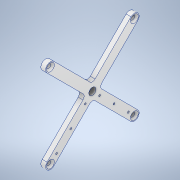
# Autodesk Inventor part: winch_support
Saved by Autodesk Inventor 2020.2 (Build 242310000, 310)
## iProperties
Created: 2020-03-23
Part Number: winch_support
Material: Aluminum 6061
Document SubType Name: Modeling
Designer: agmle
Density: 2.7 g/cm^3
Appearance: Aluminum - Flat
Mass: 66.4597 g
Surface Area: 128.224 cm^2
Volume: 24.6147 cm^3
Author: agmle
Autodesk Inventor part; units mm, degrees
ref_plane "YZ Plane" through (0, 0, 0) normal (1, 0, 0) x (0, 1, 0)
ref_plane "XZ Plane" through (0, 0, 0) normal (0, 1, 0) x (-1, 0, 0)
ref_plane "XY Plane" through (0, 0, 0) normal (0, 0, 1) x (1, 0, 0)
sketch "Sketch1" plane through (0, 0, 0) normal (1, 0, 0) x (0, 1, 0)
  arc A0 (60.1677, 51.1875) -> (51.1875, 60.1677) centre (55.6776, 55.6776) ccw
  arc A1 (51.1875, -60.1677) -> (60.1677, -51.1875) centre (55.6776, -55.6776) ccw
  arc A2 (-60.1677, -51.1875) -> (-51.1875, -60.1677) centre (-55.6776, -55.6776) ccw
  arc A3 (-51.1875, 60.1677) -> (-60.1677, 51.1875) centre (-55.6776, 55.6776) ccw
  line L0 (55.6776, 55.6776) -> (-55.6776, 55.6776) construction
  line L1 (-55.6776, 55.6776) -> (-55.6776, -55.6776) construction
  line L2 (-55.6776, -55.6776) -> (55.6776, -55.6776) construction
  line L3 (55.6776, -55.6776) -> (55.6776, 55.6776) construction
  line L4 (0, 8.9803) -> (0, -8.9803) construction
  line L5 (51.1875, 60.1677) -> (0, 8.9803)
  line L6 (-8.9803, 0) -> (-60.1677, -51.1875)
  line L7 (60.1677, -51.1875) -> (8.9803, 0)
  line L8 (0, 8.9803) -> (-51.1875, 60.1677)
  line L9 (60.1677, 51.1875) -> (8.9803, 0)
  line L10 (0, -8.9803) -> (-51.1875, -60.1677)
  line L11 (-60.1677, 51.1875) -> (-8.9803, 0)
  line L12 (0, -8.9803) -> (51.1875, -60.1677)
  line L13 (8.9803, 0) -> (-8.9803, 0) construction
  line L14 (55.6776, 55.6776) -> (-55.6776, -55.6776) construction
  point P0 (0, 0)
  point P1 (0, 0)
  dimension "d0" = 6.35
  dimension "d1" = 157.48
  constraints: 30 end point, 13 tangent, 8 point on circle, 5 coincident, 4 centre point, 3 equal radius, 3 parallel, 2 midpoint, 2 perpendicular, 1 horizontal
  measures "d0" radius of A0
  measures "d1" distance of L1.end L0.start
extrude "Extrusion1" add sketch "Sketch1" along normal blind 6.35
sketch "Sketch2" plane through (6.35, 0, 0) normal (1, 0, 0) x (0, 0, -1)
  arc A0 (-51.1875, 60.1677) -> (-60.1677, 51.1875) centre (-55.6776, 55.6776) ccw construction
  arc A1 (60.1677, 51.1875) -> (51.1875, 60.1677) centre (55.6776, 55.6776) ccw construction
  arc A2 (51.1875, -60.1677) -> (60.1677, -51.1875) centre (55.6776, -55.6776) ccw construction
  arc A3 (-60.1677, -51.1875) -> (-51.1875, -60.1677) centre (-55.6776, -55.6776) ccw construction
  point P0 (0, 0)
  constraints: 4 coincident
hole "Hole1" at (6.35, 55.6776, 55.6776) at (6.35, 55.6776, -55.6776) at (6.35, -55.6776, -55.6776) at (6.35, -55.6776, 55.6776) direction (-1, 0, 0) diameter 5.5118 end through all countersink diameter 10.3886 countersink angle 90 clearance for "Flat Head Machine Screw" size "M5" standard "Ansi Metric M Profile"
hole "Hole2" at (0, 0, 0) direction (1, 0, 0) diameter 9.525 end through all
fillet "Fillet1" radius 5 4 edges at (3.175, 8.9803, 0) (3.175, 0, -8.9803) (3.175, 0, 8.9803) (3.175, -8.9803, 0)
sketch "Sketch5" plane through (6.35, 0, 0) normal (1, 0, 0) x (0, 0, -1)
  circle A0 centre (0, 0) radius 6.35 construction
  line L0 (60.1677, -51.1875) -> (12.5158, -3.5355) construction
  circle A1 centre (-55.6776, -55.6776) radius 2.7559 construction
  line L1 (-55.6776, -55.6776) -> (0, 0) construction
  circle A2 centre (55.6776, -55.6776) radius 2.7559 construction
  line L2 (0, 0) -> (55.6776, -55.6776) construction
  line L3 (-9.525, -9.525) -> (9.525, -9.525) construction
  line L4 (28.575, -28.575) -> (-28.575, -28.575) construction
  line L5 (-47.625, -47.625) -> (47.625, -47.625) construction
  line L6 (0, -47.625) -> (0, -28.575) construction
  line L7 (0, -28.575) -> (0, -9.525) construction
  dimension "d24" = 3.175
  dimension "d25" = 19.05
  constraints: 14 end point, 6 point on line, 3 midpoint, 2 collinear, 1 centre point, 1 coincident, 1 horizontal, 1 parallel, 1 perpendicular, 1 tangent
  measures "d24" distance edge to line of A0 L3
  measures "d25" distance of L6.end L7.end
hole "Hole3" at (6.35, -47.625, 47.625) at (6.35, -28.575, 28.575) at (6.35, -9.525, 9.525) at (6.35, -9.525, -9.525) at (6.35, -28.575, -28.575) at (6.35, -47.625, -47.625) direction (-1, 0, 0) diameter 2.459 end through all thread size "M3x0.5" class "6H" standard "ANSI Metric M Profile"
body "Solid1"
